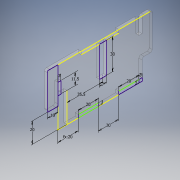
# Autodesk Inventor part: cham_right_v2
Saved by Autodesk Inventor 2017.2 (Build 212233000, 233)
## iProperties
Created: 2017-06-09
Part Number: cham_right_v2
Material: Generic
Document SubType Name: Modeling
Designer: SandeepSH
Density: 1 g/cm^3
Appearance: Polycarbonate - Clear
Author: SandeepSH
Autodesk Inventor part; units mm, degrees
ref_plane "YZ Plane" through (0, 0, 0) normal (1, 0, 0) x (0, 1, 0)
ref_plane "XZ Plane" through (0, 0, 0) normal (0, 1, 0) x (-1, 0, 0)
ref_plane "XY Plane" through (0, 0, 0) normal (0, 0, 1) x (1, 0, 0)
sketch "Sketch1" plane through (0, 0, 0) normal (1, 0, 0) x (0, 1, 0)
  line L0 (0, 0) -> (55.5, 0)
  line L1 (55.5, 0) -> (55.5, -83)
  line L2 (55.5, -83) -> (0, -83)
  line L3 (0, -83) -> (0, 0)
  dimension "d0" = 55.5
  dimension "d1" = 83
  constraints: 8 end point, 2 parallel, 1 horizontal, 1 perpendicular
  measures "d0" distance of L1.end L2.end
  measures "d1" distance of L0.end L1.end
extrude "Extrusion1" add sketch "Sketch1" along normal blind 3
sketch "Sketch2" plane through (3, 0, 0) normal (1, 0, 0) x (0, 0, -1)
  line L0 (20, 0) -> (40, 0)
  line L1 (40, 0) -> (40, 3)
  line L2 (40, 3) -> (20, 3)
  line L3 (20, 3) -> (20, 0)
  line L4 (0, 55.5) -> (0, 0) projected
  line L5 (0, 0) -> (83, 0) projected
  line L6 (60, 0) -> (80, 0)
  line L7 (80, 0) -> (80, 3)
  line L8 (80, 3) -> (60, 3)
  line L9 (60, 3) -> (60, 0)
  line L10 (83, 0) -> (80, 0)
  line L11 (80, 0) -> (80, 3)
  line L12 (80, 3) -> (83, 3)
  line L13 (83, 3) -> (83, 0)
  dimension "d4" = 20
  dimension "d5" = 3
  dimension "d6" = 20
  dimension "d7" = 20
  dimension "d8" = 20
  dimension "d11" = 3
  dimension "d12" = 3
  constraints: 24 end point, 6 parallel, 3 horizontal, 3 perpendicular, 1 point on line
  measures "d4" distance of L2.end L1.end
  measures "d5" distance of L1.end L0.end
  measures "d6" distance between parallel lines of L3 L4
  measures "d7" distance of L8.end L7.end
  measures "d8" distance between parallel lines of L9 L1
  measures "d11" distance of L11.end L12.end
  measures "d12" distance of L10.end L11.end
extrude "Extrusion2" cut sketch "Sketch2" against normal through all contours L3 L2 L1 L0 | L9 L8 L7 L5
extrude "Extrusion3" cut sketch "Sketch2" against normal through all contours L7 L12 L13 L5
sketch "Sketch3" plane through (3, 0, 0) normal (1, 0, 0) x (0, 0, -1)
  point P0 (0, 0)
sketch "Sketch4" plane through (3, 0, 0) normal (1, 0, 0) x (0, 0, -1)
  point P0 (0, 0)
sketch "Sketch5" plane through (3, 0, 0) normal (1, 0, 0) x (0, 0, -1)
  line L0 (0, 0) -> (0, 55.5) projected
  line L1 (0, 55.5) -> (-10, 55.5)
  line L2 (-10, 55.5) -> (-10, 20)
  line L3 (-10, 20) -> (0, 20)
  line L4 (0, 20) -> (0, 55.5)
  line L5 (0, 0) -> (20, 0) projected
  line L6 (83, 55.5) -> (93, 55.5)
  line L7 (93, 55.5) -> (93, 20)
  line L8 (93, 20) -> (83, 20)
  line L9 (83, 20) -> (83, 55.5)
  dimension "d15" = 10
  dimension "d16" = 20
  dimension "d28" = 10
  dimension "d29" = 20
  constraints: 16 end point, 4 parallel, 2 horizontal, 2 perpendicular
  measures "d15" distance of L3.end L2.end
  measures "d16" distance between parallel lines of L5 L3
  measures "d28" distance between parallel lines of L7 L9
  measures "d29" distance between parallel lines of L5 L8
extrude "Extrusion6" add sketch "Sketch5" against normal blind 3 contours L6 L7 L8 L9
fillet "Fillet1" radius 2 3 edges at (1.5, 55.5, -93) (1.5, 20, -93) (1.5, 20, -83) curvature continuous yes
sketch "Sketch7" plane through (3, 0, 0) normal (1, 0, 0) x (0, 0, -1)
  point P0 (0, 0)
sketch "Sketch8" plane through (3, 0, 0) normal (1, 0, 0) x (0, 0, -1)
  line L0 (0, 55.5) -> (0, 0) projected
  line L1 (0, 0) -> (9, 0)
  line L2 (9, 0) -> (9, 29)
  line L3 (9, 29) -> (0, 29)
  line L4 (0, 29) -> (0, 0)
  dimension "d33" = 9
  dimension "d34" = 29
  constraints: 8 end point, 2 parallel, 1 horizontal, 1 perpendicular
  measures "d33" distance of L3.end L2.end
  measures "d34" distance of L2.end L1.end
extrude "Extrusion7" cut sketch "Sketch8" against normal through all
sketch "Sketch9" plane through (3, 0, 0) normal (1, 0, 0) x (0, 0, -1)
  line L0 (0, 55.5) -> (91, 55.5) projected
  line L1 (0, 55.5) -> (-10, 55.5)
  line L2 (-10, 55.5) -> (-10, 20)
  line L3 (-10, 20) -> (0, 20)
  line L4 (0, 20) -> (0, 55.5)
  line L5 (9, 0) -> (20, 0) projected
  point P0 (0, 0)
  dimension "d37" = 10
  dimension "d39" = 20
  constraints: 8 end point, 2 parallel, 1 horizontal, 1 perpendicular
  measures "d37" distance of L3.end L2.end
  measures "d39" distance between parallel lines of L5 L3
extrude "Extrusion8" add sketch "Sketch9" against normal blind 3
sketch "Sketch10" plane through (3, 0, 0) normal (1, 0, 0) x (0, 0, -1)
  line L0 (0, 29) -> (0, 20) projected
  line L1 (0, 29) -> (3, 29)
  line L2 (3, 29) -> (3, 40.5)
  line L3 (3, 40.5) -> (0, 40.5)
  line L4 (0, 40.5) -> (0, 29)
  point P0 (0, 0)
  dimension "d42" = 3
  dimension "d43" = 11.5
  constraints: 8 end point, 2 parallel, 1 horizontal, 1 perpendicular
  measures "d42" distance of L3.end L2.end
  measures "d43" distance of L2.end L1.end
extrude "Extrusion9" cut sketch "Sketch10" against normal through all
fillet "Fillet2" radius 2 4 edges at (1.5, 20, 10) (1.5, 20, 0) (1.5, 29, -3) (1.5, 55.5, 10) curvature continuous yes
sketch "Sketch11" plane through (3, 0, 0) normal (1, 0, 0) x (0, 0, -1)
  line L0 (-8, 55.5) -> (91, 55.5) projected
  line L1 (80, 55.5) -> (83, 55.5)
  line L2 (83, 55.5) -> (83, 40.5)
  line L3 (83, 40.5) -> (80, 40.5)
  line L4 (80, 40.5) -> (80, 55.5)
  line L5 (93, 53.5) -> (93, 22) projected
  point P0 (0, 0)
  dimension "d47" = 3
  dimension "d48" = 15
  dimension "d49" = 10
  constraints: 8 end point, 2 parallel, 1 horizontal, 1 perpendicular, 1 point on line
  measures "d47" distance of L2.end L3.end
  measures "d48" distance of L1.end L2.end
  measures "d49" distance between parallel lines of L5 L2
extrude "Extrusion10" cut sketch "Sketch11" against normal through all
fillet "Fillet3" radius 2 2 edges at (1.5, 55.5, -80) (1.5, 55.5, -83) curvature continuous yes
sketch "Sketch12" plane through (3, 0, 0) normal (1, 0, 0) x (0, 0, -1)
  line L0 (-8, 55.5) -> (78, 55.5) projected
  line L1 (23, 55.5) -> (60, 55.5)
  line L2 (60, 55.5) -> (60, 52.5)
  line L3 (60, 52.5) -> (23, 52.5)
  line L4 (23, 52.5) -> (23, 55.5)
  line L5 (80, 40.5) -> (80, 53.5) projected
  line L6 (3, 40.5) -> (3, 31) projected
  point P0 (0, 0)
  dimension "d53" = 3
  dimension "d54" = 20
  dimension "d55" = 20
  constraints: 8 end point, 2 parallel, 1 horizontal, 1 perpendicular, 1 point on line
  measures "d53" distance of L1.end L2.end
  measures "d54" distance between parallel lines of L5 L2
  measures "d55" distance between parallel lines of L4 L6
extrude "Extrusion11" cut sketch "Sketch12" against normal through all
sketch "Sketch13" plane through (3, 0, 0) normal (1, 0, 0) x (0, 0, -1)
  line L0 (23, 52.5) -> (60, 52.5) projected
  line L1 (41, 52.5) -> (48, 52.5)
  line L2 (48, 52.5) -> (48, 22.5)
  line L3 (48, 22.5) -> (41, 22.5)
  line L4 (41, 22.5) -> (41, 52.5)
  line L5 (0, 55.5) -> (0, 0) projected
  line L6 (9, 29) -> (9, 0) projected
  point P0 (44.5, 22.5)
  dimension "d58" = 7
  dimension "d59" = 30
  dimension "d63" = 35.5
  constraints: 8 end point, 2 parallel, 1 horizontal, 1 midpoint, 1 perpendicular, 1 point on line
  measures "d58" distance of L2.end L3.end
  measures "d59" distance of L1.end L2.end
  measures "d63" distance from line of L6 point (44.5, 22.5)
extrude "Extrusion12" cut sketch "Sketch13" against normal through all
equation "\"d6\" = d4"
equation "\"d28\" = d15"
equation "\"d29\" = d16"
body "Solid1"
